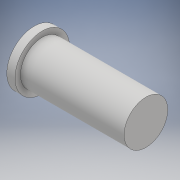
# Autodesk Inventor part: Circuit_MJ165H
Saved by Autodesk Inventor 2018 (Build 220112000, 112)
## iProperties
Created: 2018-02-15
Part Number: Circuit_MJ165H
Material: 一般
Document SubType Name: Modeling
Designer: sktom
Density: 1 g/cm^3
Appearance: 既定
Author: sktom
Autodesk Inventor part; units mm, degrees
ref_plane "YZ Plane" through (0, 0, 0) normal (1, 0, 0) x (0, 1, 0)
ref_plane "XZ Plane" through (0, 0, 0) normal (0, 1, 0) x (-1, 0, 0)
ref_plane "XY Plane" through (0, 0, 0) normal (0, 0, 1) x (1, 0, 0)
sketch "スケッチ1" plane through (0, 0, 0) normal (0, 0, 1) x (1, 0, 0)
  line L0 (0, 0) -> (0, 5)
  line L1 (0, 5) -> (1.5, 5)
  line L2 (1.5, 5) -> (1.5, 4)
  line L3 (1.5, 4) -> (20.5, 4)
  line L4 (20.5, 4) -> (20.5, 0)
  line L5 (20.5, 0) -> (0, 0)
  dimension "d0" = 5
  dimension "d1" = 1.5
  dimension "d2" = 4
  dimension "d3" = 20.5
  constraints: 12 end point, 5 perpendicular, 1 vertical
  measures "d0" distance of L0.start L0.end
  measures "d1" distance of L0.end L1.end
  measures "d2" distance between parallel lines of L5 L3
  measures "d3" distance between parallel lines of L0 L4
revolve "回転1" add sketch "スケッチ1" angle 360 about axis through (20.5, 0, 0) along (-1, 0, 0)
sketch "スケッチ2" plane through (0, 0, 0) normal (-1, 0, 0) x (0, 0, 1)
  circle A0 centre (0, 0) radius 1.25
  dimension "d5" = 2.5
  constraints: 1 centre point, 1 coincident
  measures "d5" diameter of A0
extrude "押し出し1" cut sketch "スケッチ2" against normal blind 15
